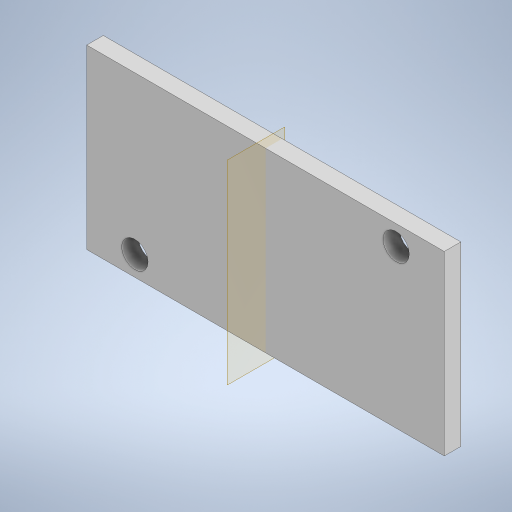
# Autodesk Inventor part: V3-buck-din-rail-mount
Saved by Autodesk Inventor 2023 (Build 270158030, 158C)
## iProperties
Created: 2024-03-29
Part Number: V3-buck-din-rail-mount
Material: Generic
Document SubType Name: Modeling
Designer: Imogen Heard
Density: 1 g/cm^3
Appearance: Default
Author: Imogen Heard
Autodesk Inventor part; units mm, degrees
ref_plane "XZ Plane" through (0, 0, 0) normal (0, 1, 0) x (-1, 0, 0)
ref_plane "XY Plane" through (0, 0, 0) normal (0, 0, 1) x (1, 0, 0)
sketch "DIN-rail-mount" plane through (0, 0, 0) normal (0, 0, 1) x (1, 0, 0)
  line L0 (-33.7324, 10.3063) -> (-34.1071, 10.3063)
  arc A0 (-34.1071, 10.3063) -> (-34.0972, 8.9045) centre (-34.0349, 9.6059) ccw
  line L1 (-34.0972, 8.9045) -> (-34.0972, 7.5962)
  line L2 (-34.0972, 7.5962) -> (-10.5472, 7.5962)
  line L3 (-15.1777, 10.5962) -> (-10.5472, 10.5962)
  spline S0 degree 4 poles (-15.1777, 10.5962) (-16.8449, 11.2147) (-17.4384, 12.1609) (-17.614, 13.5609) (-17.8782, 16.561) (-19.4782, 17.121) (-20.5125, 16.6872) (-20.0803, 14.0765) (-19.9141, 11.8671) (-20.831, 11.2147) (-21.1411, 10.8766) (-21.3946, 10.7087) (-21.5869, 10.5962) knots -3 -3 -3 -3 -3 -2.876473 -2.236311 -2 -1.83789 -1.739488 -1.512977 -1.110527 -1.050464 -1 -1 -1 -1 -1
  line L4 (-15.1777, 10.5962) -> (-16.8449, 11.2147) construction
  line L5 (-16.8449, 11.2147) -> (-17.4384, 12.1609) construction
  line L6 (-17.4384, 12.1609) -> (-17.614, 13.5609) construction
  line L7 (-17.614, 13.5609) -> (-17.8782, 16.561) construction
  line L8 (-17.8782, 16.561) -> (-19.4782, 17.121) construction
  line L9 (-19.4782, 17.121) -> (-20.5125, 16.6872) construction
  line L10 (-20.5125, 16.6872) -> (-20.0803, 14.0765) construction
  line L11 (-20.0803, 14.0765) -> (-19.9141, 11.8671) construction
  line L12 (-19.9141, 11.8671) -> (-20.831, 11.2147) construction
  line L13 (-20.831, 11.2147) -> (-21.1411, 10.8766) construction
  line L14 (-21.1411, 10.8766) -> (-21.3946, 10.7087) construction
  line L15 (-21.3946, 10.7087) -> (-21.5869, 10.5962) construction
  line L16 (-21.5869, 10.5962) -> (-28.3279, 10.5962)
  spline S1 degree 4 poles (-28.3279, 10.5962) (-28.3774, 11.1364) (-28.3774, 12.1962) (-27.4303, 11.8538) (-27.3668, 11.5141) (-27.2583, 13.8149) (-27.5062, 15.5334) (-29.0652, 16.1148) (-31.2529, 16.2494) (-33.2894, 16.2494) (-35.6023, 15.8436) (-38.121, 14.7599) (-38.8386, 12.0503) (-37.1134, 10.3122) (-35.7126, 9.8375) (-35.0159, 10.5962) (-35.5227, 12.1898) (-36.6765, 12.025) (-37.0094, 13.5091) (-35.0159, 13.9186) (-34.2446, 13.0997) (-34.1909, 11.9608) (-33.793, 10.5076) (-33.7324, 10.3063) knots -17.993985 -17.993985 -17.993985 -17.993985 -17.993985 -16.993985 -15.993985 -14.993985 -13.993985 -12.993985 -11.993985 -10.993985 -9.993985 -8.993985 -7.993985 -6.993985 -5.993985 -4.993985 -3.993985 -2.993985 -2.159505 -1.993985 -1.73171 -1.02637 -1 -1 -1 -1 -1
  line L17 (-28.3279, 10.5962) -> (-28.3774, 11.1364) construction
  line L18 (-28.3774, 11.1364) -> (-28.3774, 12.1962) construction
  line L19 (-28.3774, 12.1962) -> (-27.4303, 11.8538) construction
  line L20 (-27.4303, 11.8538) -> (-27.3668, 11.5141) construction
  line L21 (-27.3668, 11.5141) -> (-27.2583, 13.8149) construction
  line L22 (-27.2583, 13.8149) -> (-27.5062, 15.5334) construction
  line L23 (-27.5062, 15.5334) -> (-29.0652, 16.1148) construction
  line L24 (-29.0652, 16.1148) -> (-31.2529, 16.2494) construction
  line L25 (-31.2529, 16.2494) -> (-33.2894, 16.2494) construction
  line L26 (-33.2894, 16.2494) -> (-35.6023, 15.8436) construction
  line L27 (-35.6023, 15.8436) -> (-38.121, 14.7599) construction
  line L28 (-38.121, 14.7599) -> (-38.8386, 12.0503) construction
  line L29 (-38.8386, 12.0503) -> (-37.1134, 10.3122) construction
  line L30 (-37.1134, 10.3122) -> (-35.7126, 9.8375) construction
  line L31 (-35.7126, 9.8375) -> (-35.0159, 10.5962) construction
  line L32 (-35.0159, 10.5962) -> (-35.5227, 12.1898) construction
  line L33 (-33.793, 10.5076) -> (-33.7324, 10.3063) construction
  spline S2 degree 4 poles (-33.2324, 10.5924) (-33.2773, 11.299) (-33.4667, 13.0378) (-33.1081, 14.1456) (-31.1461, 14.939) (-29.7454, 14.4515) (-29.2931, 13.6814) (-28.9087, 13.027) (-28.682, 12.025) (-28.7279, 10.6) knots -6.977977 -6.977977 -6.977977 -6.977977 -6.977977 -6 -5 -4 -3 -2 -1 -1 -1 -1 -1
  line L34 (-33.2324, 10.5924) -> (-33.2773, 11.299) construction
  line L35 (-33.2773, 11.299) -> (-33.4667, 13.0378) construction
  line L36 (-33.4667, 13.0378) -> (-33.1081, 14.1456) construction
  line L37 (-33.1081, 14.1456) -> (-31.1461, 14.939) construction
  line L38 (-31.1461, 14.939) -> (-29.7454, 14.4515) construction
  line L39 (-29.7454, 14.4515) -> (-29.2931, 13.6814) construction
  line L40 (-29.2931, 13.6814) -> (-28.9087, 13.027) construction
  line L41 (-28.9087, 13.027) -> (-28.682, 12.025) construction
  line L42 (-28.682, 12.025) -> (-28.7279, 10.6) construction
  line L43 (-28.7279, 10.6) -> (-29.5316, 10.5924)
  spline S3 degree 4 poles (-29.5316, 10.5924) (-29.7743, 11.7709) (-30.187, 13.195) (-31.4721, 13.572) (-32.387, 13.1292) (-32.387, 11.4703) (-32.4859, 10.5924) knots -4 -4 -4 -4 -4 -3 -2 -1 -1 -1 -1 -1
  line L44 (-29.5316, 10.5924) -> (-29.7743, 11.7709) construction
  line L45 (-29.7743, 11.7709) -> (-30.187, 13.195) construction
  line L46 (-30.187, 13.195) -> (-31.4721, 13.572) construction
  line L47 (-31.4721, 13.572) -> (-32.387, 13.1292) construction
  line L48 (-32.387, 13.1292) -> (-32.387, 11.4703) construction
  line L49 (-32.387, 11.4703) -> (-32.4859, 10.5924) construction
  line L50 (-32.4859, 10.5924) -> (-33.2324, 10.5924)
  line L51 (-10.5472, 10.5962) -> (-10.5472, 7.5962)
  line L52 (-35.5227, 12.1898) -> (-36.6765, 12.025) construction
  line L53 (-36.6765, 12.025) -> (-37.0094, 13.5091) construction
  line L54 (-37.0094, 13.5091) -> (-35.0159, 13.9186) construction
  line L55 (-35.0159, 13.9186) -> (-34.2446, 13.0997) construction
  line L56 (-34.2446, 13.0997) -> (-34.1909, 11.9608) construction
  line L57 (-34.1909, 11.9608) -> (-33.793, 10.5076) construction
  point P0 (-10.1883, 12.0835)
  point P1 (-29.1297, 10.5962)
  point P2 (-10.5472, 9.0962)
  dimension "d41" = 23.55
  dimension "d43" = 3
  dimension "d44" = 0.4
  dimension "d45" = 17.7807
  dimension "d46" = 4.6306
  dimension "d47" = 6.4092
  dimension "d48" = 0.9179
  dimension "d49" = 1.2576
  dimension "d50" = 1.6
  dimension "d51" = 0.8037
  dimension "d52" = 2.9543
  dimension "d53" = 0.7465
  dimension "d54" = 0.5
  dimension "d117" = 3
  dimension "d123" = 16.8196
  dimension "d124" = 17.8302
  dimension "d125" = 16.7111
  dimension "d126" = 0.7041
  dimension "d127" = 93.521
  dimension "d129" = 4.3709
  dimension "d130" = 0.2899
  dimension "d131" = 0.0038
  dimension "d132" = 18.5181
  dimension "d133" = 20.7057
  dimension "d137" = 23.4877
  dimension "d138" = 0.9904
  measures "d41" distance between parallel lines of L1 L51
  measures "d43" distance between parallel lines of L2 L16
  measures "d44" distance of L42.end L16.end
  measures "d45" distance from line of L16.end L51
  measures "d46" distance from line of L51 L3.start
  measures "d47" distance of L16.start L3.start
  measures "d48" distance from line of L16 L20.end
  measures "d49" distance from line of L16 L19.end
  measures "d50" distance from line of L16 L18.end
  measures "d51" distance of L43.end L42.end
  measures "d52" distance of L49.end L43.end
  measures "d53" distance of L34.start L49.end
  measures "d54" horizontal distance of L33.end L34.start
  measures "d117" distance between parallel lines of L2 L3
  measures "d123" horizontal distance of point (-10.547, 9.096) L20.end
  measures "d124" distance from line of L51 L17.end
  measures "d125" distance from line of L51 L21.end
  measures "d126" radius of A0
  measures "d127" angle of L24 L51
  measures "d129" distance from line of L3.end L24
  measures "d130" distance from line of L3.end L0
  measures "d131" distance from line of L42.end L3
  measures "d132" distance from line of L23.end L51
  measures "d133" distance from line of L24.end L51
  measures "d137" distance from line of A0.centre L51
  measures "d138" distance from line of A0.centre L3
sketch "Sketch1" plane through (0, 0, 0) normal (0, 0, 1) x (1, 0, 0)
  line L0 (-21.5, 10.6) -> (21.5, 10.6) projected
  line L1 (-21.5, -10.6) -> (-21.5, 10.6) projected
  line L2 (21.5, -10.6) -> (-21.5, -10.6) projected
  line L3 (21.5, 10.6) -> (21.5, -10.6) projected
  circle A0 centre (-15.78, -8.3) radius 1.59 projected
  circle A1 centre (15.78, 8.3) radius 1.59 projected
  line L4 (-21.6, -10.7) -> (-21.6, 10.7)
  line L5 (-21.6, 10.7) -> (21.6, 10.7)
  line L6 (21.6, 10.7) -> (21.6, -10.7)
  line L7 (21.6, -10.7) -> (-21.6, -10.7)
  point P0 (0, 0)
  dimension "d167" = 0.1
  constraints: 8 end point, 3 other
  measures "d167" distance between parallel lines of L2 L7
extrude "Extrusion1" add sketch "Sketch1" against normal blind 2 contours L0 L3 L2 L1 | L4 L5 L6 L7
ref_plane "Work Plane1" through (0, 0, 0) normal (0, 0, 1) x (1, 0, 0)
sketch "Sketch2" plane through (0, -10.6, 0) normal (0, 1, 0) x (1, 0, 0)
  line L0 (-21.5, 0) -> (21.5, 0) projected
  line L1 (-21.5, 0) -> (-21.5, 2) projected
  line L2 (21.5, 2) -> (-21.5, 2) projected
  line L3 (21.5, 0) -> (21.5, 2) projected
  line L4 (-21.5, 0) -> (21.5, 0) projected
  line L5 (-23.1852, 2.7101) -> (-23.56, 2.7101)
  arc A0 (-23.56, 2.7101) -> (-23.55, 1.3083) centre (-23.4877, 2.0096) ccw
  line L6 (-23.55, 1.3083) -> (-23.55, 0)
  line L7 (-23.55, 0) -> (0, 0)
  line L8 (-4.6306, 3) -> (0, 3)
  spline S0 degree 4 poles (-4.6306, 3) (-6.2977, 3.6185) (-6.8912, 4.5646) (-7.0668, 5.9647) (-7.331, 8.9647) (-8.9311, 9.5248) (-9.9653, 9.0909) (-9.5331, 6.4802) (-9.3669, 4.2709) (-10.2838, 3.6185) (-10.5939, 3.2804) (-10.8475, 3.1125) (-11.0397, 3) knots -3 -3 -3 -3 -3 -2.876473 -2.236311 -2 -1.83789 -1.739488 -1.512977 -1.110527 -1.050464 -1 -1 -1 -1 -1
  line L9 (-4.6306, 3) -> (-6.2977, 3.6185) construction
  line L10 (-6.2977, 3.6185) -> (-6.8912, 4.5646) construction
  line L11 (-6.8912, 4.5646) -> (-7.0668, 5.9647) construction
  line L12 (-7.0668, 5.9647) -> (-7.331, 8.9647) construction
  line L13 (-7.331, 8.9647) -> (-8.9311, 9.5248) construction
  line L14 (-8.9311, 9.5248) -> (-9.9653, 9.0909) construction
  line L15 (-9.9653, 9.0909) -> (-9.5331, 6.4802) construction
  line L16 (-9.5331, 6.4802) -> (-9.3669, 4.2709) construction
  line L17 (-9.3669, 4.2709) -> (-10.2838, 3.6185) construction
  line L18 (-10.2838, 3.6185) -> (-10.5939, 3.2804) construction
  line L19 (-10.5939, 3.2804) -> (-10.8475, 3.1125) construction
  line L20 (-10.8475, 3.1125) -> (-11.0397, 3) construction
  line L21 (-11.0397, 3) -> (-17.7807, 3)
  spline S1 degree 4 poles (-17.7807, 3) (-17.8302, 3.5402) (-17.8302, 4.6) (-16.8831, 4.2576) (-16.8196, 3.9179) (-16.7111, 6.2186) (-16.9591, 7.9372) (-18.5181, 8.5185) (-20.7057, 8.6531) (-22.7423, 8.6531) (-25.0552, 8.2473) (-27.5738, 7.1636) (-28.2915, 4.4541) (-26.5662, 2.716) (-25.1655, 2.2413) (-24.4688, 3) (-24.9756, 4.5936) (-26.1293, 4.4288) (-26.4622, 5.9129) (-24.4688, 6.3224) (-23.6974, 5.5034) (-23.6438, 4.3645) (-23.2459, 2.9114) (-23.1852, 2.7101) knots -17.993985 -17.993985 -17.993985 -17.993985 -17.993985 -16.993985 -15.993985 -14.993985 -13.993985 -12.993985 -11.993985 -10.993985 -9.993985 -8.993985 -7.993985 -6.993985 -5.993985 -4.993985 -3.993985 -2.993985 -2.159505 -1.993985 -1.73171 -1.02637 -1 -1 -1 -1 -1
  line L22 (-17.7807, 3) -> (-17.8302, 3.5402) construction
  line L23 (-17.8302, 3.5402) -> (-17.8302, 4.6) construction
  line L24 (-17.8302, 4.6) -> (-16.8831, 4.2576) construction
  line L25 (-16.8831, 4.2576) -> (-16.8196, 3.9179) construction
  line L26 (-16.8196, 3.9179) -> (-16.7111, 6.2186) construction
  line L27 (-16.7111, 6.2186) -> (-16.9591, 7.9372) construction
  line L28 (-16.9591, 7.9372) -> (-18.5181, 8.5185) construction
  line L29 (-18.5181, 8.5185) -> (-20.7057, 8.6531) construction
  line L30 (-20.7057, 8.6531) -> (-22.7423, 8.6531) construction
  line L31 (-22.7423, 8.6531) -> (-25.0552, 8.2473) construction
  line L32 (-25.0552, 8.2473) -> (-27.5738, 7.1636) construction
  line L33 (-27.5738, 7.1636) -> (-28.2915, 4.4541) construction
  line L34 (-28.2915, 4.4541) -> (-26.5662, 2.716) construction
  line L35 (-26.5662, 2.716) -> (-25.1655, 2.2413) construction
  line L36 (-25.1655, 2.2413) -> (-24.4688, 3) construction
  line L37 (-24.4688, 3) -> (-24.9756, 4.5936) construction
  line L38 (-23.2459, 2.9114) -> (-23.1852, 2.7101) construction
  spline S2 degree 4 poles (-22.6852, 2.9962) (-22.7301, 3.7028) (-22.9196, 5.4416) (-22.5609, 6.5494) (-20.5989, 7.3428) (-19.1982, 6.8553) (-18.7459, 6.0852) (-18.3615, 5.4308) (-18.1349, 4.4288) (-18.1807, 3.0038) knots -6.977977 -6.977977 -6.977977 -6.977977 -6.977977 -6 -5 -4 -3 -2 -1 -1 -1 -1 -1
  line L39 (-22.6852, 2.9962) -> (-22.7301, 3.7028) construction
  line L40 (-22.7301, 3.7028) -> (-22.9196, 5.4416) construction
  line L41 (-22.9196, 5.4416) -> (-22.5609, 6.5494) construction
  line L42 (-22.5609, 6.5494) -> (-20.5989, 7.3428) construction
  line L43 (-20.5989, 7.3428) -> (-19.1982, 6.8553) construction
  line L44 (-19.1982, 6.8553) -> (-18.7459, 6.0852) construction
  line L45 (-18.7459, 6.0852) -> (-18.3615, 5.4308) construction
  line L46 (-18.3615, 5.4308) -> (-18.1349, 4.4288) construction
  line L47 (-18.1349, 4.4288) -> (-18.1807, 3.0038) construction
  line L48 (-18.1807, 3.0038) -> (-18.9844, 2.9962)
  spline S3 degree 4 poles (-18.9844, 2.9962) (-19.2271, 4.1746) (-19.6398, 5.5988) (-20.9249, 5.9758) (-21.8399, 5.533) (-21.8399, 3.874) (-21.9387, 2.9962) knots -4 -4 -4 -4 -4 -3 -2 -1 -1 -1 -1 -1
  line L49 (-18.9844, 2.9962) -> (-19.2271, 4.1746) construction
  line L50 (-19.2271, 4.1746) -> (-19.6398, 5.5988) construction
  line L51 (-19.6398, 5.5988) -> (-20.9249, 5.9758) construction
  line L52 (-20.9249, 5.9758) -> (-21.8399, 5.533) construction
  line L53 (-21.8399, 5.533) -> (-21.8399, 3.874) construction
  line L54 (-21.8399, 3.874) -> (-21.9387, 2.9962) construction
  line L55 (-21.9387, 2.9962) -> (-22.6852, 2.9962)
  line L56 (0, 3) -> (0, 0)
  line L57 (-24.9756, 4.5936) -> (-26.1293, 4.4288) construction
  line L58 (-26.1293, 4.4288) -> (-26.4622, 5.9129) construction
  line L59 (-26.4622, 5.9129) -> (-24.4688, 6.3224) construction
  line L60 (-24.4688, 6.3224) -> (-23.6974, 5.5034) construction
  line L61 (-23.6974, 5.5034) -> (-23.6438, 4.3645) construction
  line L62 (-23.6438, 4.3645) -> (-23.2459, 2.9114) construction
  point P0 (-22.7633, 3)
  point P1 (-18.4291, 3)
  point P2 (-19.1408, 3)
  point P3 (-22.095, 3)
  point P4 (-4.5838, 3)
  point P5 (-11.055, 3)
  point P6 (-17.6386, 3)
  point P7 (-23.4853, 3)
  point P8 (-23.4853, 2.7)
  point P9 (-23.4853, 1.3)
  point P10 (-23.4853, 0)
  point P11 (0, 2)
  point P12 (0, 0)
  point P13 (0, 0)
  constraints: 2 midpoint, 2 other
extrude "Extrusion2" [suppressed]
mirror "Mirror1" [suppressed]
extrude "Extrusion6" [suppressed]
sketch "Sketch6" plane through (-17.7807, -10.6, -3) normal (0, -1, 0) x (1, 0, 0)
  line L0 (-2.7693, 1) -> (38.2307, 1)
  line L1 (38.2307, 1) -> (38.2307, 20.5)
  line L2 (38.2307, 20.5) -> (-2.7693, 20.5)
  line L3 (-2.7693, 20.5) -> (-2.7693, 1)
  line L4 (-5.7693, 3) -> (41.3307, 3) projected
  line L5 (-5.7693, 1.6917) -> (-5.7693, 3) projected
  line L6 (41.3307, 1.6917) -> (41.3307, 3) projected
  point P0 (41.3307, 2.3459)
  dimension "d149" = 17.5
  dimension "d150" = 41
  dimension "d151" = 3
  dimension "d152" = 3.1
  dimension "d153" = 2
  constraints: 8 end point, 2 parallel, 1 horizontal, 1 midpoint, 1 perpendicular
  measures "d149" distance between parallel lines of L2 L4
  measures "d150" distance between parallel lines of L1 L3
  measures "d151" distance between parallel lines of L5 L3
  measures "d152" distance from line of point (41.331, 2.346) L1
  measures "d153" distance between parallel lines of L4 L0
extrude "Extrusion16" [suppressed]
sketch "Sketch8" plane through (-17.7807, -10.6, -3) normal (0, 1, 0) x (1, 0, 0)
  line L0 (30.2307, -6) -> (5.2307, -6)
  line L1 (5.2307, -6) -> (5.2307, -3)
  line L2 (5.2307, -3) -> (30.2307, -3)
  line L3 (30.2307, -3) -> (30.2307, -6)
  line L4 (-2.7693, -20.5) -> (-2.7693, -3) projected
  line L5 (38.2307, -3) -> (38.2307, -20.5) projected
  dimension "d156" = 8
  dimension "d157" = 8
  dimension "d158" = 3
  constraints: 8 end point, 2 parallel, 1 horizontal, 1 perpendicular
  measures "d156" distance between parallel lines of L4 L1
  measures "d157" distance between parallel lines of L3 L5
  measures "d158" distance between parallel lines of L0 L2
extrude "Extrusion8" [suppressed]
mirror "Mirror2" [suppressed]
sketch "Sketch9" plane through (-21.5, 10.6, 17.5) normal (0, 0, 1) x (1, 0, 0)
  line L0 (41.95, 0) -> (0.95, 0) projected
  line L1 (41.95, 0) -> (41.95, 2) projected
  line L2 (41.95, 2) -> (0.95, 2) projected
  line L3 (0.95, 0) -> (0.95, 2) projected
extrude "Extrusion9" [suppressed]
ref_plane "Work Plane10" through (-12.55, 10.6, 4.3) normal (0, 0, 1) x (1, 0, 0)
sketch "Sketch12" plane through (-12.55, -10.6, 4.3) normal (0, 0, 1) x (1, 0, 0)
  circle A0 centre (0, 22.2) radius 2
  circle A1 centre (25, 22.2) radius 2
  line L0 (-8, 21.2) -> (-8, 23.2) projected
  line L1 (33, 21.2) -> (-8, 21.2) projected
  line L2 (33, 23.2) -> (33, 21.2) projected
  line L3 (-8, 23.2) -> (33, 23.2) projected
  point P0 (-8, 22.2)
  point P1 (33, 22.2)
  point P2 (1.7321, 23.2)
  point P3 (-1.7321, 23.2)
  point P4 (26.7321, 23.2)
  point P5 (23.2679, 23.2)
  dimension "d76" = 4
  dimension "d164" = 8
  dimension "d165" = 8
  constraints: 2 centre point, 1 equal radius, 1 horizontal alignment
  measures "d76" diameter of A1
  measures "d164" distance of point (-8, 22.2) A0.centre
  measures "d165" distance of point (33, 22.2) A1.centre
extrude "Extrusion11" [suppressed]
sketch "Sketch13" plane through (-17.7807, -10.6, -3) normal (0, -1, 0) x (1, 0, 0)
  line L0 (-2.7693, 1) -> (-2.7693, 3) projected
  line L1 (-5.7693, 3) -> (-2.7693, 3) projected
  line L2 (-5.7693, 1.6917) -> (-5.7693, 3) projected
  arc A0 (-5.7693, 1.6917) -> (-5.7792, 0.2899) centre (-5.707, 0.9904) ccw projected
  line L3 (-5.4045, 0.2899) -> (-5.7792, 0.2899) projected
  line L4 (6.741, 0) -> (0, 0) projected
  line L5 (13.1501, 0) -> (22.4113, 0) projected
  line L6 (28.8205, 0) -> (35.5615, 0) projected
  line L7 (40.9659, 0.2899) -> (41.3407, 0.2899) projected
  arc A1 (41.3407, 0.2899) -> (41.3307, 1.6917) centre (41.2685, 0.9904) ccw projected
  line L8 (41.3307, 1.6917) -> (41.3307, 3) projected
  line L9 (38.2307, 3) -> (41.3307, 3) projected
  line L10 (38.2307, 3) -> (38.2307, 1) projected
  line L11 (38.2307, 1) -> (-2.7693, 1) projected
  line L12 (39.7194, 0.0038) -> (40.4659, 0.0038) projected
  line L13 (35.9614, -0.0038) -> (36.7651, 0.0038) projected
  line L14 (-0.4, -0.0038) -> (-1.2037, 0.0038) projected
  line L15 (-4.158, 0.0038) -> (-4.9045, 0.0038) projected
  constraints: 4 horizontal alignment, 4 other
extrude "Extrusion12" [suppressed]
mirror "Mirror3" [suppressed]
sketch "Sketch14" plane through (-17.7807, -10.6, -3) normal (0, 1, 0) x (1, 0, 0)
  line L0 (-2.7693, -10.5) -> (38.2307, -10.5) projected
  line L1 (38.2307, -1) -> (38.2307, -10.5) projected
  line L2 (-2.7693, -1) -> (38.2307, -1) projected
  line L3 (-2.7693, -10.5) -> (-2.7693, -1) projected
  line L4 (3.4987, -7.3) -> (6.9628, -7.3) projected
  line L5 (28.4987, -7.3) -> (31.9628, -7.3) projected
  line L6 (5.2307, -6) -> (5.2307, -3) projected
  line L7 (-2.7693, -3) -> (5.2307, -3) projected
  line L8 (-2.7693, -20.5) -> (-2.7693, -3) projected
  line L9 (38.2307, -20.5) -> (-2.7693, -20.5) projected
  line L10 (38.2307, -3) -> (38.2307, -20.5) projected
  line L11 (30.2307, -3) -> (38.2307, -3) projected
  line L12 (30.2307, -3) -> (30.2307, -6) projected
  line L13 (30.2307, -6) -> (5.2307, -6) projected
  point P0 (-2.7693, -10.5)
  constraints: 2 horizontal alignment
extrude "Extrusion13" [suppressed]
chamfer "Chamfer5" [suppressed]
chamfer "Chamfer6" [suppressed]
chamfer "Chamfer7" [suppressed]
ref_plane "Work Plane5" through (-15.5, 10.6, 3) normal (0, 0, 1) x (1, 0, 0)
sketch "Sketch15" plane through (-15.5, 10.6, 3) normal (0, 0, 1) x (1, 0, 0)
  line L0 (-6, -0.1356) -> (37, -0.1356)
  line L1 (37, -0.1356) -> (37, -21.1356)
  line L2 (37, -21.1356) -> (-6, -21.1356)
  line L3 (-6, -21.1356) -> (-6, -0.1356)
  dimension "d97" = 21
  dimension "d98" = 43
  constraints: 8 end point, 2 parallel, 1 horizontal, 1 perpendicular
  measures "d97" distance between parallel lines of L2 L0
  measures "d98" distance between parallel lines of L3 L1
extrude "Extrusion14" add sketch "Sketch15" along normal blind 1.3 separate body
sketch "Sketch16" plane through (-17.7807, -12.6, -3) normal (0, -1, 0) x (1, 0, 0)
  line L0 (5.2307, 3) -> (-2.7693, 3) projected
  line L1 (-2.7693, 3) -> (-5.7693, 3)
  line L2 (-5.7693, 3) -> (-5.7693, 7.3)
  line L3 (-5.7693, 7.3) -> (-2.7693, 7.3)
  line L4 (-2.7693, 7.3) -> (-2.7693, 3)
  point P0 (17.7807, 3)
  dimension "d166" = 4.3
  constraints: 8 end point, 2 parallel, 1 horizontal, 1 perpendicular
  measures "d166" distance between parallel lines of L1 L3
extrude "Extrusion15" [suppressed]
chamfer "Chamfer9" [suppressed]
chamfer "Chamfer10" [suppressed]
chamfer "Chamfer11" [suppressed]
body "Solid1"
